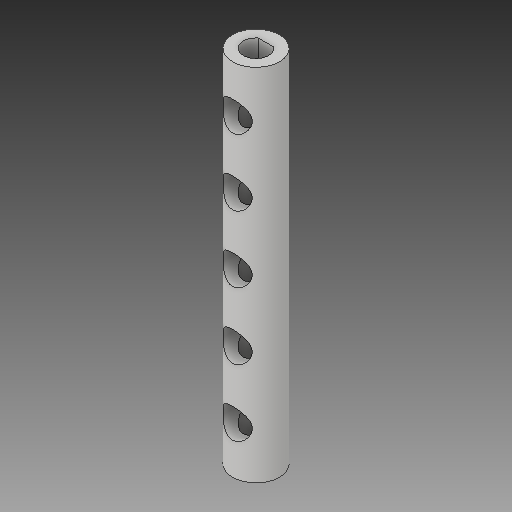
# Autodesk Inventor part: Spinner98mmDShaft
Saved by Autodesk Inventor 2019 (Build 230136000, 136)
## iProperties
Created: 2018-11-08
Part Number: Spinner98mmDShaft
Material: Generic
Document SubType Name: Modeling
Designer: Ashley
Density: 1 g/cm^3
Appearance: Default
Author: Ashley
Autodesk Inventor part; units mm, degrees
ref_plane "YZ Plane" through (0, 0, 0) normal (1, 0, 0) x (0, 1, 0)
ref_plane "XZ Plane" through (0, 0, 0) normal (0, 1, 0) x (-1, 0, 0)
sketch "Shaft Sketch" plane through (0, 0, 0) normal (0, 1, 0) x (-1, 0, 0)
  circle A0 centre (0, 0.05) radius 6
  circle A1 centre (0, 0.05) radius 6
  arc A2 (2.0149, -2.5) -> (-2.0149, -2.5) centre (0, 0.05) ccw
  line L0 (2.0149, -2.5) -> (-2.0149, -2.5)
  point P0 (0, 3.0022)
  dimension "d0" = 12
  dimension "d1" = 6.5
  dimension "d3" = 2.55
  constraints: 3 centre point, 2 coincident, 2 end point, 2 point on circle, 1 horizontal
  measures "d0" diameter of A0
  measures "d1" diameter of A2
  measures "d3" distance from line of point (0, 0.05) L0
extrude "Shaft Extrusion" add sketch "Shaft Sketch" along normal blind 92
ref_plane "Tangent" through (0, 0, -5.95) normal (0, 0, 1) x (1, 0, 0)
sketch "Holes Sketch" plane through (0, 0, -5.95) normal (0, 0, 1) x (1, 0, 0)
  line L0 (0, 112.8875) -> (0, -22.05) construction
  line L1 (44.45, 46) -> (-58.7375, 46) construction
  line L2 (6, 92) -> (-6, 92) projected
  line L3 (-6, 0) -> (6, 0) projected
  circle A0 centre (0, 46) radius 3.75
  circle A1 centre (0, 29) radius 3.75
  circle A2 centre (0, 12) radius 3.75
  circle A3 centre (0, 63) radius 3.75
  circle A4 centre (0, 46) radius 3.75
  circle A5 centre (0, 29) radius 3.75
  circle A6 centre (0, 80) radius 3.75
  circle A7 centre (0, 63) radius 3.75
  circle A8 centre (0, 46) radius 3.75
  point P0 (0, 0)
  dimension "d6" = 46
  dimension "d7" = 46
  dimension "d9" = 7.5
  dimension "d12" = 17
  dimension "d15" = 17
  constraints: 9 centre point, 4 end point, 3 vertical, 2 point on line, 1 horizontal, 16 other
  measures "d6" distance between parallel lines of L1 L2
  measures "d7" distance between parallel lines of L3 L1
  measures "d9" diameter of A0
  measures "d12" distance of A0.centre A1.centre
  measures "d15" distance of A0.centre A3.centre
extrude "Extrusion2" cut sketch "Holes Sketch" along normal through all
body "Solid1"
